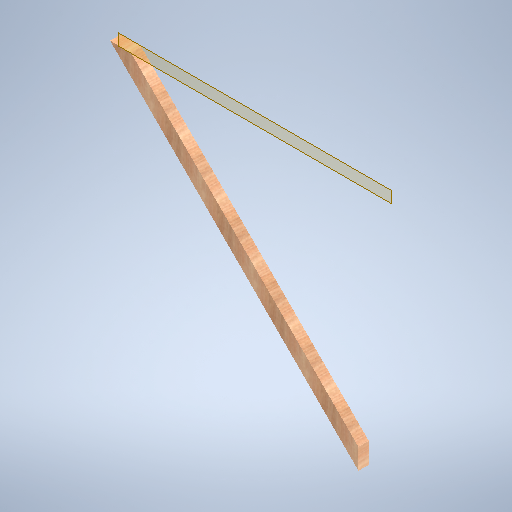
# Autodesk Inventor part: 2x4x67.88
Saved by Autodesk Inventor 2025 (Build 290162000, 162)
## iProperties
Created: 2024-09-03
Part Number: 2x4x67.88
Material: Wood (Birch)
Document SubType Name: Modeling
Designer: Win
Density: 0.55 g/cm^3
Appearance: Birch - Natural Polished
Author: Win
Autodesk Inventor part; units mm, degrees
ref_plane "YZ Plane" through (0, 0, 0) normal (1, 0, 0) x (0, 1, 0)
ref_plane "XZ Plane" through (0, 0, 0) normal (0, 1, 0) x (-1, 0, 0)
ref_plane "XY Plane" through (0, 0, 0) normal (0, 0, 1) x (1, 0, 0)
ref_plane "Work Plane1" through (0, 0, 0) normal (0, 0, 1) x (1, 0, 0)
sketch "Sketch1" plane through (0, 0, 0) normal (0, 0, 1) x (1, 0, 0)
  line L0 (0, 0) -> (-101.6, 0)
  line L1 (-101.6, 0) -> (1065.8333, -1167.4333)
  line L2 (1065.8333, -1167.4333) -> (1117.6006, -1219.2006)
  line L3 (1117.6006, -1219.2006) -> (1117.6006, -1117.6006)
  line L4 (1117.6006, -1117.6006) -> (0, 0)
  dimension "d1" = 101.6
  dimension "d2" = 1651
  dimension "d4" = 101.6
  constraints: 10 end point, 1 horizontal, 1 parallel
  measures "d1" distance of L0.start L0.end
  measures "d2" distance of L0.end L1.end
  measures "d4" distance of L2.end L3.end
extrude "Extrusion1" add sketch "Sketch1" against normal blind 50.8
body "Solid1"
